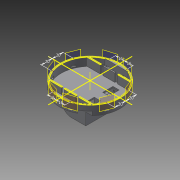
# Autodesk Inventor part: base
Saved by Autodesk Inventor 2014 (Build 180170000, 170)
## iProperties
Created: 2013-06-26
Part Number: base
Material: Generisch
Document SubType Name: Modeling
Designer: hanse
Density: 1 g/cm^3
Appearance: Vorgabe
Author: hanse
Autodesk Inventor part; units mm, degrees
ref_plane "YZ Plane" through (0, 0, 0) normal (1, 0, 0) x (0, 1, 0)
ref_plane "XZ Plane" through (0, 0, 0) normal (0, 1, 0) x (-1, 0, 0)
ref_plane "XY Plane" through (0, 0, 0) normal (0, 0, 1) x (1, 0, 0)
sketch "Skizze1" plane through (0, 0, 0) normal (0, 0, 1) x (1, 0, 0)
  line L0 (29, -20.75) -> (-29, -20.75) projected
  line L1 (29, 20.75) -> (29, -20.75) projected
  line L2 (-29, 20.75) -> (29, 20.75) projected
  line L3 (-29, -20.75) -> (-29, 20.75) projected
  line L4 (4, 34.75) -> (14, 34.75) projected
  line L5 (40.5, 34.75) -> (14, 34.75) projected
  line L6 (14, -34.75) -> (40.5, -34.75) projected
  line L7 (14, -34.75) -> (4, -34.75) projected
  line L8 (40.5, -34.75) -> (40.5, -21.05) projected
  line L9 (40.5, -21.05) -> (40.5, -7.75) projected
  line L10 (40.5, 21.05) -> (40.5, 7.75) projected
  line L11 (40.5, 34.75) -> (40.5, 21.05) projected
  line L12 (4, 34.75) -> (4, 21.05)
  line L13 (4, -34.75) -> (4, -21.05)
  line L14 (13.5, 17.844) -> (13.5, 38.186)
  line L15 (13.5, -17.844) -> (13.5, -38.186)
  line L16 (0, 0) -> (29, 0)
  line L17 (13.5, 17.844) -> (13.5, -17.844)
  line L18 (-15.5, 46.05) -> (42.5, 46.05) projected
  line L19 (42.5, 38.05) -> (-15.5, 38.05) projected
  line L20 (-15.5, -38.05) -> (42.5, -38.05) projected
  line L21 (42.5, -46.05) -> (-15.5, -46.05) projected
  circle A0 centre (13.5, 0) radius 55
  line L22 (40.5, -7.75) -> (29, -7.75)
  line L23 (29, -7.75) -> (29, -26.5586)
  line L24 (29, -26.5586) -> (40.5, -26.5586)
  line L25 (40.5, -26.5586) -> (40.5, -7.75)
  line L26 (40.5, 7.75) -> (40.5, 26.6995)
  line L27 (40.5, 26.6995) -> (29, 26.6995)
  line L28 (29, 26.6995) -> (29, 7.75)
  line L29 (40.5, 7.75) -> (38.25, 7.75) projected
  line L30 (38.25, 7.75) -> (31.25, 7.75) projected
  line L31 (31.25, 7.75) -> (29, 7.75) projected
  line L32 (40.5, 7.75) -> (29, 7.75)
  line L33 (-27.4199, 36.75) -> (54.4199, 36.75)
  line L34 (-27.4199, -36.75) -> (54.4199, -36.75)
  dimension "d0" = 2
  dimension "d1" = 2
  dimension "d22" = 110
  constraints: 32 end point, 5 parallel, 4 point on circle, 4 vertical, 3 collinear, 3 point on line, 2 midpoint, 2 perpendicular, 1 centre point, 1 horizontal, 6 other
  measures "d0" distance between parallel lines of L5 L33
  measures "d1" distance between parallel lines of L6 L34
  measures "d22" diameter of A0
ref_plane "Arbeitsebene1" through (30, 21.05, 2.35) normal (0, 0, 1) x (1, 0, 0)
extrude "Extrusion1" add sketch "Skizze1" along normal up to surface (2.35 mm away) contours L23 L24 L8 L6 L7 L15 L0 | L0 L15 L17 L16 L1 | L15 L34 A0 L33 L14 L2 L3 L0 | L0 L3 L2 L14 L17 L15 | L1 L31 L30 L29 L10 L11 L5 L4 L14 L33 A0 L34 L15 L7 L6 L8 L9 L22 | L16 L17 L14 L2 L1 | L14 L4 L5 L11 L27 L28 L2
sketch "Skizze2" plane through (0, 0, 0) normal (0, 0, -1) x (-1, 0, 0)
  line L0 (-29, 26.6995) -> (-29, 7.75) projected
  line L1 (-29, 7.75) -> (-40.5, 7.75) projected
  line L2 (-40.5, 7.75) -> (-40.5, 26.6995) projected
  line L3 (-40.5, 26.6995) -> (-29, 26.6995) projected
  line L4 (-40.5, -26.5586) -> (-40.5, -7.75) projected
  line L5 (-40.5, -7.75) -> (-29, -7.75) projected
  line L6 (-29, -7.75) -> (-29, -26.5586) projected
  line L7 (-29, -26.5586) -> (-40.5, -26.5586) projected
  line L8 (-54.4199, 36.75) -> (27.4199, 36.75) projected
  line L9 (27.4199, -36.75) -> (-54.4199, -36.75) projected
  line L10 (-29, -20.75) -> (29, -20.75) projected
  line L11 (29, 20.75) -> (-29, 20.75) projected
  line L12 (-42.5, 36.75) -> (-42.5, -36.75)
  line L13 (-29, 7.75) -> (-29, -7.75)
  line L14 (1, 36.75) -> (1, 20.75)
  line L15 (1, -20.75) -> (1, -36.75)
  line L16 (-4, 34.75) -> (-4, 21.05)
  line L17 (-4, -34.75) -> (-4, -21.05)
  point P0 (0, 0)
  dimension "d4" = 2
  dimension "d5" = 5
  constraints: 12 end point, 6 point on line, 3 perpendicular, 2 collinear, 2 vertical, 4 other
  measures "d4" distance between parallel lines of L2 L12
  measures "d5" distance between parallel lines of L14 L16
ref_plane "Arbeitsebene2" through (14, 21.05, -20) normal (0, 0, -1) x (0, 1, 0)
extrude "Extrusion2" add sketch "Skizze2" along normal up to surface (20 mm away) contours L3 L2 L1 L13 L5 L4 L7 L6 L10 L15 L9 L12 L8 L14 L11 L0
sketch "Skizze3" plane through (-1, 20.75, 0) normal (0, -1, 0) x (1, 0, 0)
  line L0 (0, -20) -> (30, -20) projected
  line L1 (30, 0) -> (30, -20) projected
  line L2 (0, 0) -> (30, 0) projected
  line L3 (30, -20) -> (41.5, -20) projected
  line L4 (41.5, -20) -> (30, -20)
  line L5 (30, -20) -> (30, 0)
  line L6 (30, 0) -> (41.5, 0)
  line L7 (41.5, 0) -> (41.5, -20)
  arc A0 (15, 0) -> (15, -20) centre (15, -10) ccw projected
  point P0 (1, 0)
  constraints: 8 end point, 2 parallel, 1 horizontal, 1 perpendicular
ref_plane "Arbeitsebene3" through (4, 34.75, -20) normal (0, 1, 0) x (0, 0, 1)
extrude "Extrusion3" cut sketch "Skizze3" against normal up to surface (14 mm away) contours L1 L6 L7 L3
sketch "Skizze4" plane through (14, 34.75, 0) normal (0, -1, 0) x (1, 0, 0)
  circle A0 centre (8.9, -11.9) radius 1.5 projected
  circle A1 centre (-0.5, -10) radius 2.5 projected
  circle A2 centre (15.5, -6.5) radius 1.5 projected
  point P0 (-14, 0)
extrude "Extrusion4" cut sketch "Skizze4" against normal blind 0.5
sketch "Skizze5" plane through (14, 34.75, -20) normal (0, -1, 0) x (1, 0, 0)
  circle A0 centre (-0.5, 10) radius 1.5 projected
  point P0 (-14, 20)
extrude "Extrusion5" cut sketch "Skizze5" against normal through all
mirror "Spiegeln1" about plane through (0, 0, 0) normal (0, 1, 0) of "Extrusion5", "Extrusion3"
sketch "Skizze6" plane through (14, -34.75, 0) normal (0, 1, 0) x (1, 0, 0)
  circle A0 centre (15.5, 13.5) radius 1.5 projected
  circle A1 centre (8.9, 8.1) radius 1.5 projected
  circle A2 centre (-0.5, 10) radius 2.5 projected
  point P0 (-14, 0)
extrude "Extrusion6" cut sketch "Skizze6" against normal blind 0.5
sketch "Skizze7" plane through (42.5, 36.75, -20) normal (0, 0, -1) x (-1, 0, 0)
  line L0 (43.5, -73.5) -> (0, -73.5)
  line L1 (0, -73.5) -> (0, 0)
  line L2 (0, 0) -> (43.5, 0)
  line L3 (43.5, 0) -> (43.5, -73.5)
  point P0 (42.5, -36.75)
  constraints: 8 end point, 2 parallel, 1 horizontal, 1 perpendicular
extrude "Extrusion7" add sketch "Skizze7" along normal blind 2
sketch "Skizze8" plane through (42.5, 36.75, -22) normal (0, 0, -1) x (-1, 0, 0)
  line L0 (43.5, -73.5) -> (43.5, 0) projected
  line L1 (71.5, -16) -> (13.5, -16) projected
  line L2 (13.5, -57.5) -> (71.5, -57.5) projected
  line L3 (13.5, -16) -> (43.5, -16)
  line L4 (43.5, -16) -> (43.5, -57.5)
  line L5 (43.5, -57.5) -> (13.5, -57.5)
  line L6 (13.5, -57.5) -> (13.5, -16)
  line L7 (11.25, -12.5) -> (11.25, -29) projected
  line L8 (4.25, -29) -> (11.25, -29) projected
  line L9 (4.25, -12.5) -> (4.25, -29) projected
  line L10 (11.25, -12.5) -> (4.25, -12.5) projected
  line L11 (11.25, -61) -> (4.25, -61) projected
  line L12 (4.25, -61) -> (4.25, -44.5) projected
  line L13 (11.25, -44.5) -> (4.25, -44.5) projected
  line L14 (11.25, -61) -> (11.25, -44.5) projected
  line L15 (13.5, -44.5) -> (13.5, -63.3086) projected
  line L16 (13.5, -63.3086) -> (2, -63.3086) projected
  line L17 (2, -63.3086) -> (2, -44.5) projected
  line L18 (2, -44.5) -> (13.5, -44.5) projected
  line L19 (2, -10.0505) -> (13.5, -10.0505) projected
  line L20 (13.5, -10.0505) -> (13.5, -29) projected
  line L21 (13.5, -29) -> (2, -29) projected
  line L22 (2, -29) -> (2, -10.0505) projected
  point P0 (42.5, -36.75)
  constraints: 8 end point, 2 parallel, 2 point on line, 1 horizontal, 1 perpendicular
extrude "Extrusion8" cut sketch "Skizze8" against normal up to next
fillet "Rundung1" radius 17 2 edges at (-1, 28.75, -22) (-1, -28.75, -22)
sketch "Skizze9" plane through (-27.4199, 36.75, 2.35) normal (0, 0, 1) x (1, 0, 0)
  line L0 (0, 0) -> (81.8398, 0) projected
  arc A0 (0, 0) -> (0, -73.5) centre (40.9199, -36.75) ccw projected
  line L1 (81.8398, -73.5) -> (0, -73.5) projected
  arc A1 (81.8398, -73.5) -> (81.8398, 0) centre (40.9199, -36.75) ccw projected
  arc A2 (0.9019, -2) -> (0.9019, -71.5) centre (40.9199, -36.75) ccw
  line L2 (0.9019, -2) -> (80.9379, -2)
  arc A3 (80.9379, -71.5) -> (80.9379, -2) centre (40.9199, -36.75) ccw
  line L3 (80.9379, -71.5) -> (0.9019, -71.5)
  line L4 (0, 0) -> (0, -3.0667)
  line L5 (0, -70.4333) -> (0, -73.5)
  line L6 (81.8398, -73.5) -> (81.8398, -70.4333)
  line L7 (81.8398, 0) -> (81.8398, -3.0667)
  line L8 (0, -2) -> (81.8398, -2)
  line L9 (0, -71.5) -> (81.8398, -71.5)
  circle A4 centre (40.9199, -36.75) radius 55
  line L10 (11.9199, 9.3) -> (69.9199, 9.3) projected
  line L11 (69.9199, -82.8) -> (11.9199, -82.8) projected
  line L12 (15.0762, -85.3) -> (66.7636, -85.3)
  line L13 (15.0762, 11.8) -> (66.7636, 11.8)
  point P0 (27.4199, -36.75)
  dimension "d23" = 2
  dimension "d24" = 2
  dimension "d25" = 2
  dimension "d140" = 2.5
  dimension "d141" = 2.5
  constraints: 20 end point, 12 point on circle, 4 perpendicular, 4 point on line, 3 centre point, 2 equal length, 2 horizontal, 1 coincident, 1 concentric, 3 other
  measures "d23" radial gap between concentric circles of A0 A2
  measures "d24" distance between parallel lines of L9 L1
  measures "d25" distance between parallel lines of L8 L0
  measures "d140" distance between parallel lines of L10 L13
  measures "d141" distance between parallel lines of L11 L12
extrude "Extrusion9" add sketch "Skizze9" along normal blind 5 contours L4 A2 L5 A0 | L0 L7 L8 L2 L4 | A1 L6 A3 L7 | L5 L9 L3 L6 L1 | A4 L13 | L12 A4
sketch "Skizze11" plane through (-27.4199, 36.75, 7.35) normal (0, 0, 1) x (1, 0, 0)
  line L0 (0, -2) -> (81.8398, -2) projected
  line L1 (81.8398, -2) -> (81.8398, -3.0667) projected
  arc A0 (81.8398, -70.4333) -> (81.8398, -3.0667) centre (40.9199, -36.75) ccw projected
  line L2 (81.8398, -70.4333) -> (81.8398, -71.5) projected
  line L3 (81.8398, -71.5) -> (0, -71.5) projected
  line L4 (0, -71.5) -> (0, -70.4333) projected
  arc A1 (0, -3.0667) -> (0, -70.4333) centre (40.9199, -36.75) ccw projected
  line L5 (0, -3.0667) -> (0, -2) projected
  arc A2 (0, 0) -> (0, -73.5) centre (40.9199, -36.75) ccw projected
  line L6 (0, -73.5) -> (81.8398, -73.5) projected
  arc A3 (81.8398, -73.5) -> (81.8398, 0) centre (40.9199, -36.75) ccw projected
  line L7 (81.8398, 0) -> (0, 0) projected
  circle A4 centre (40.9199, -36.75) radius 53
  circle A5 centre (40.9199, -36.75) radius 55
  line L8 (15.0762, 11.8) -> (66.7636, 11.8) projected
  line L9 (66.7636, -85.3) -> (15.0762, -85.3) projected
  line L10 (19.662, 11.8) -> (62.1778, 11.8)
  line L11 (62.1778, -85.3) -> (19.662, -85.3)
  point P0 (27.4199, -36.75)
  constraints: 5 point on circle, 4 end point, 4 point on line, 2 coincident, 1 centre point, 3 other
extrude "Extrusion11" add sketch "Skizze11" along normal blind 10 contours L5 A1 L4 L3 A4 L6 A2 L7 L0 | A4 L7 L0 | A4 L7 A3 L6 L3 L2 A0 L1 L0 | L7 A5 L8 A4 | A4 L8 A5 L7 | L8 A5 A4 | L3 A4 L6 | L6 A4 L9 A5 | L9 A4 A5 | L6 A5 L9 A4
sketch "Skizze23" plane through (-27.4199, 36.75, 7.35) normal (0, 0, 1) x (1, 0, 0)
  arc A0 (19.662, -85.3) -> (62.1778, -85.3) centre (40.9199, -36.75) ccw projected
  line L0 (62.1778, -85.3) -> (19.662, -85.3) projected
  arc A1 (62.1778, 11.8) -> (19.662, 11.8) centre (40.9199, -36.75) ccw projected
  line L1 (19.662, 11.8) -> (62.1778, 11.8) projected
  point P0 (27.4199, -36.75)
extrude "Extrusion19" add sketch "Skizze23" along normal up to surface (10 mm away)
sketch "Skizze12" plane through (13.5, 0, 17.35) normal (0, 0, 1) x (1, 0, 0)
  line L0 (-38.1895, 36.75) -> (38.1895, 36.75) projected
  line L1 (40.9199, -34.75) -> (-40.9199, -34.75) projected
  line L2 (-40.9199, -34.75) -> (-40.9199, -33.6833) projected
  arc A0 (-40.9199, 33.6833) -> (-40.9199, -33.6833) centre (0, 0) ccw projected
  line L3 (-40.9199, 33.6833) -> (-40.9199, 34.75) projected
  line L4 (-40.9199, 34.75) -> (40.9199, 34.75) projected
  line L5 (40.9199, 34.75) -> (40.9199, 33.6833) projected
  arc A1 (40.9199, -33.6833) -> (40.9199, 33.6833) centre (0, 0) ccw projected
  line L6 (40.9199, -33.6833) -> (40.9199, -34.75) projected
  line L7 (-15.9199, 34.75) -> (-15.9199, 36.75)
  line L8 (-15.9199, 36.75) -> (-10.9199, 36.75)
  line L9 (-10.9199, 36.75) -> (-10.9199, 34.75)
  line L10 (-10.9199, 34.75) -> (-15.9199, 34.75)
  line L11 (15.9199, 36.75) -> (10.9199, 36.75)
  line L12 (10.9199, 36.75) -> (10.9199, 34.75)
  line L13 (15.9199, 34.75) -> (10.9199, 34.75)
  line L14 (15.9199, 34.75) -> (15.9199, 36.75)
  point P0 (-13.5, 0)
  dimension "d158" = 25
  dimension "d159" = 25
  dimension "d160" = 5
  dimension "d161" = 5
  constraints: 16 end point, 8 point on line, 4 perpendicular, 2 collinear
  measures "d158" distance between parallel lines of L7 L3
  measures "d159" distance between parallel lines of L14 L5
  measures "d160" distance of L9.end L7.start
  measures "d161" distance of L11.start L11.end
extrude "Extrusion12" cut sketch "Skizze12" against normal up to surface (15 mm away) contours L0 L9 L4 L7 | L4 L5 A1 L6 L1 L2 A0 L3 | L0 L14 L4 L12
mirror "Spiegeln2" about plane through (0, 0, 0) normal (0, 1, 0) of "Extrusion12"
sketch "Skizze13" plane through (13.5, 0, 17.35) normal (0, 0, 1) x (1, 0, 0)
  line L0 (15.9199, -34.75) -> (15.9199, -36.75) projected
  line L1 (38.1895, -36.75) -> (15.9199, -36.75) projected
  arc A0 (-38.1895, -36.75) -> (38.1895, -36.75) centre (0, 0) ccw projected
  line L2 (-15.9199, -36.75) -> (-38.1895, -36.75) projected
  line L3 (-15.9199, -36.75) -> (-15.9199, -34.75) projected
  line L4 (-15.9199, -34.75) -> (-40.9199, -34.75) projected
  line L5 (-40.9199, -34.75) -> (-40.9199, -33.6833) projected
  arc A1 (-40.9199, 33.6833) -> (-40.9199, -33.6833) centre (0, 0) ccw projected
  line L6 (-40.9199, 33.6833) -> (-40.9199, 34.75) projected
  line L7 (-40.9199, 34.75) -> (-15.9199, 34.75) projected
  line L8 (-15.9199, 34.75) -> (-15.9199, 36.75) projected
  line L9 (-38.1895, 36.75) -> (-15.9199, 36.75) projected
  arc A2 (38.1895, 36.75) -> (-38.1895, 36.75) centre (0, 0) ccw projected
  line L10 (15.9199, 36.75) -> (38.1895, 36.75) projected
  line L11 (15.9199, 36.75) -> (15.9199, 34.75) projected
  line L12 (15.9199, 34.75) -> (40.9199, 34.75) projected
  line L13 (40.9199, 34.75) -> (40.9199, 33.6833) projected
  arc A3 (40.9199, -33.6833) -> (40.9199, 33.6833) centre (0, 0) ccw projected
  line L14 (40.9199, -33.6833) -> (40.9199, -34.75) projected
  line L15 (40.9199, -34.75) -> (15.9199, -34.75) projected
  circle A4 centre (0, 0) radius 55 projected
  line L16 (0, 77) -> (0, -77) projected
  line L17 (-77, 0) -> (77, 0) projected
  line L18 (-48.4401, -18.9091) -> (-51.2348, -20)
  line L19 (48.4401, 18.9091) -> (51.2348, 20)
  line L20 (49.3717, -19.2727) -> (51.2348, -20)
  line L21 (-51.2348, 20) -> (-49.3717, 19.2727)
  line L22 (-16, -52.6213) -> (-15.4182, -50.7078)
  line L23 (16, -52.6213) -> (15.4182, -50.7078)
  line L24 (15.4182, 50.7078) -> (16, 52.6213)
  line L25 (-15.4182, 50.7078) -> (-16, 52.6213)
  line L26 (10.9199, -36.75) -> (10.9199, -34.75) projected
  line L27 (10.9199, -34.75) -> (-10.9199, -34.75) projected
  line L28 (-10.9199, -34.75) -> (-10.9199, -36.75) projected
  line L29 (10.9199, -36.75) -> (-10.9199, -36.75) projected
  point P0 (-13.5, 0)
  dimension "d42" = 20
  dimension "d65" = 20
  dimension "d70" = 20
  dimension "d77" = 20
  dimension "d78" = 16
  dimension "d79" = 16
  dimension "d88" = 16
  dimension "d89" = 16
  constraints: 16 end point, 6 point on circle, 5 line through centre, 12 other
  measures "d42" distance from line of L17 L18.end
  measures "d65" distance from line of L17 L19.end
  measures "d70" distance from line of L17 L20.end
  measures "d77" distance from line of L17 L21.start
  measures "d78" distance from line of L25.end L16
  measures "d79" distance from line of L16 L24.end
  measures "d88" distance from line of L16 L22.start
  measures "d89" distance from line of L16 L23.start
ref_plane "Arbeitsebene4" through (-37.7348, -20, 17.35) normal (-0.931541, -0.3636364, 0) x (0.3636364, -0.931541, 0)
ref_plane "Arbeitsebene5" through (-37.7348, 20, 17.35) normal (-0.931541, 0.3636364, 0) x (-0.3636364, -0.931541, 0)
ref_plane "Arbeitsebene6" through (-2.5, 52.6213, 17.35) normal (-0.2909091, 0.9567507, 0) x (-0.9567507, -0.2909091, 0)
ref_plane "Arbeitsebene7" through (29.5, 52.6213, 17.35) normal (0.2909091, 0.9567507, 0) x (-0.9567507, 0.2909091, 0)
ref_plane "Arbeitsebene8" through (64.7348, 20, 17.35) normal (0.931541, 0.3636364, 0) x (-0.3636364, 0.931541, 0)
ref_plane "Arbeitsebene9" through (64.7348, -20, 17.35) normal (0.931541, -0.3636364, 0) x (0.3636364, 0.931541, 0)
ref_plane "Arbeitsebene10" through (29.5, -52.6213, 17.35) normal (0.2909091, -0.9567507, 0) x (0.9567507, 0.2909091, 0)
ref_plane "Arbeitsebene11" through (-2.5, -52.6213, 17.35) normal (-0.2909091, -0.9567507, 0) x (0.9567507, -0.2909091, 0)
sketch "Skizze14" plane through (-37.7348, -20, 17.35) normal (-0.931541, -0.3636364, 0) x (0.3636364, -0.931541, 0)
  line L0 (16.4974, -15) -> (-46.2573, -15) projected
  line L1 (-3.75, -10) -> (3.75, -10)
  line L2 (3.75, -10) -> (3.75, -13)
  line L3 (3.75, -13) -> (-3.75, -13)
  line L4 (-3.75, -13) -> (-3.75, -10)
  line L5 (0, -15) -> (0, 15)
  point P0 (-4.9091, -17.35)
  point P1 (0, 0)
  point P2 (0, 0)
  dimension "d94" = 7.5
  dimension "d95" = 3
  dimension "d97" = 2
  dimension "d100" = 3.75
  constraints: 10 end point, 3 parallel, 1 coincident, 1 horizontal, 1 midpoint, 1 perpendicular, 1 point on line
  measures "d94" distance of L1.start L1.end
  measures "d95" distance of L1.end L2.end
  measures "d97" distance between parallel lines of L0 L3
  measures "d100" distance between parallel lines of L5 L2
extrude "Extrusion16" cut sketch "Skizze14" against normal up to next
sketch "Skizze15" plane through (-37.7348, 20, 17.35) normal (-0.931541, 0.3636364, 0) x (-0.3636364, -0.931541, 0)
  line L0 (-3.75, -10) -> (3.75, -10)
  line L1 (3.75, -10) -> (3.75, -13)
  line L2 (3.75, -13) -> (-3.75, -13)
  line L3 (-3.75, -13) -> (-3.75, -10)
  line L4 (0, -15) -> (0, 15)
  line L5 (46.2573, -15) -> (-16.4974, -15) projected
  point P0 (-6.1364, -17.35)
  point P1 (0, 0)
  point P2 (0, 0)
  dimension "d101" = 7.5
  dimension "d102" = 3
  dimension "d104" = 3.75
  dimension "d129" = 2
  constraints: 10 end point, 3 parallel, 1 coincident, 1 horizontal, 1 midpoint, 1 perpendicular
  measures "d101" distance of L0.start L0.end
  measures "d102" distance of L0.end L1.end
  measures "d104" distance between parallel lines of L4 L1
  measures "d129" distance between parallel lines of L5 L2
extrude "Extrusion17" cut sketch "Skizze15" against normal up to next
sketch "Skizze16" plane through (-2.5, 52.6213, 17.35) normal (-0.2909091, 0.9567507, 0) x (-0.9567507, -0.2909091, 0)
  line L0 (-3.75, -10) -> (3.75, -10)
  line L1 (3.75, -10) -> (3.75, -13)
  line L2 (3.75, -13) -> (-3.75, -13)
  line L3 (-3.75, -13) -> (-3.75, -10)
  line L4 (0, -15) -> (0, 15)
  line L5 (5.1223, -15) -> (29.041, -15) projected
  point P0 (-6.1364, -17.35)
  point P1 (0, 0)
  point P2 (0, 0)
  dimension "d105" = 7.5
  dimension "d106" = 3
  dimension "d108" = 3.75
  dimension "d148" = 2
  constraints: 10 end point, 3 parallel, 1 coincident, 1 horizontal, 1 midpoint, 1 perpendicular
  measures "d105" distance of L0.start L0.end
  measures "d106" distance of L0.end L1.end
  measures "d108" distance between parallel lines of L4 L1
  measures "d148" distance between parallel lines of L2 L5
sketch "Skizze17" plane through (29.5, 52.6213, 17.35) normal (0.2909091, 0.9567507, 0) x (-0.9567507, 0.2909091, 0)
  line L0 (-3.75, -10) -> (3.75, -10)
  line L1 (3.75, -10) -> (3.75, -13)
  line L2 (3.75, -13) -> (-3.75, -13)
  line L3 (-3.75, -13) -> (-3.75, -10)
  line L4 (0, -15) -> (0, 15)
  line L5 (-29.041, -15) -> (-5.1223, -15) projected
  point P0 (-6.1364, -17.35)
  point P1 (0, 0)
  point P2 (0, 0)
  dimension "d109" = 7.5
  dimension "d110" = 3
  dimension "d112" = 3.75
  dimension "d149" = 2
  constraints: 10 end point, 3 parallel, 1 coincident, 1 horizontal, 1 midpoint, 1 perpendicular
  measures "d109" distance of L0.start L0.end
  measures "d110" distance of L0.end L1.end
  measures "d112" distance between parallel lines of L4 L1
  measures "d149" distance between parallel lines of L5 L2
sketch "Skizze18" plane through (64.7348, 20, 17.35) normal (0.931541, 0.3636364, 0) x (-0.3636364, 0.931541, 0)
  line L0 (-3.75, -10) -> (3.75, -10)
  line L1 (3.75, -10) -> (3.75, -13)
  line L2 (3.75, -13) -> (-3.75, -13)
  line L3 (-3.75, -13) -> (-3.75, -10)
  line L4 (0, -15) -> (0, 15)
  line L5 (16.4974, -15) -> (-46.2573, -15) projected
  point P0 (-6.1364, -17.35)
  point P1 (0, 0)
  point P2 (0, 0)
  dimension "d113" = 7.5
  dimension "d114" = 3
  dimension "d116" = 3.75
  dimension "d131" = 2
  constraints: 10 end point, 3 parallel, 1 coincident, 1 horizontal, 1 midpoint, 1 perpendicular
  measures "d113" distance of L0.start L0.end
  measures "d114" distance of L0.end L1.end
  measures "d116" distance between parallel lines of L4 L1
  measures "d131" distance between parallel lines of L2 L5
extrude "Extrusion15" cut sketch "Skizze18" against normal up to next
sketch "Skizze19" plane through (64.7348, -20, 17.35) normal (0.931541, -0.3636364, 0) x (0.3636364, 0.931541, 0)
  line L0 (-3.75, -10) -> (3.75, -10)
  line L1 (3.75, -10) -> (3.75, -13)
  line L2 (3.75, -13) -> (-3.75, -13)
  line L3 (-3.75, -13) -> (-3.75, -10)
  line L4 (0, -15) -> (0, 15)
  line L5 (46.2573, -15) -> (-16.4974, -15) projected
  point P0 (-6.1364, -17.35)
  point P1 (0, 0)
  point P2 (0, 0)
  dimension "d117" = 7.5
  dimension "d118" = 3
  dimension "d120" = 3.75
  dimension "d130" = 2
  constraints: 10 end point, 3 parallel, 1 coincident, 1 horizontal, 1 midpoint, 1 perpendicular
  measures "d117" distance of L0.start L0.end
  measures "d118" distance of L0.end L1.end
  measures "d120" distance between parallel lines of L4 L1
  measures "d130" distance between parallel lines of L2 L5
extrude "Extrusion14" cut sketch "Skizze19" against normal up to next
sketch "Skizze20" plane through (29.5, -52.6213, 17.35) normal (0.2909091, -0.9567507, 0) x (0.9567507, 0.2909091, 0)
  line L0 (-3.75, -10) -> (3.75, -10)
  line L1 (3.75, -10) -> (3.75, -13)
  line L2 (3.75, -13) -> (-3.75, -13)
  line L3 (-3.75, -13) -> (-3.75, -10)
  line L4 (0, -15) -> (0, 15)
  line L5 (-20.5567, -15) -> (0.3385, -15) projected
  point P0 (-6.1364, -17.35)
  point P1 (0, 0)
  point P2 (0, 0)
  dimension "d121" = 7.5
  dimension "d122" = 3
  dimension "d124" = 3.75
  dimension "d146" = 2
  constraints: 10 end point, 3 parallel, 1 coincident, 1 horizontal, 1 midpoint, 1 perpendicular
  measures "d121" distance of L0.start L0.end
  measures "d122" distance of L0.end L1.end
  measures "d124" distance between parallel lines of L4 L1
  measures "d146" distance between parallel lines of L5 L2
sketch "Skizze21" plane through (-2.5, -52.6213, 17.35) normal (-0.2909091, -0.9567507, 0) x (0.9567507, -0.2909091, 0)
  line L0 (-3.75, -10) -> (3.75, -10)
  line L1 (3.75, -10) -> (3.75, -13)
  line L2 (3.75, -13) -> (-3.75, -13)
  line L3 (-3.75, -13) -> (-3.75, -10)
  line L4 (0, -15) -> (0, 15)
  line L5 (-29.041, -15) -> (-5.1223, -15) projected
  point P0 (-6.1364, -17.35)
  point P1 (0, 0)
  point P2 (0, 0)
  dimension "d125" = 7.5
  dimension "d126" = 3
  dimension "d128" = 3.75
  dimension "d147" = 2
  constraints: 10 end point, 3 parallel, 1 coincident, 1 horizontal, 1 midpoint, 1 perpendicular
  measures "d125" distance of L0.start L0.end
  measures "d126" distance of L0.end L1.end
  measures "d128" distance between parallel lines of L4 L1
  measures "d147" distance between parallel lines of L2 L5
extrude "Extrusion20" cut sketch "Skizze17" against normal up to next
extrude "Extrusion21" cut sketch "Skizze16" against normal up to next
extrude "Extrusion22" cut sketch "Skizze20" against normal up to next
extrude "Extrusion23" cut sketch "Skizze21" against normal up to next
sketch "Skizze24" plane through (0, 0, 0) normal (0, 0, -1) x (-1, 0, 0)
  line L0 (-42.5, -36.75) -> (-42.5, 36.75) projected
  arc A0 (-54.4199, 33.6833) -> (-54.4199, -33.6833) centre (-13.5, 0) ccw projected
  line L1 (-54.4199, 33.6833) -> (-54.4199, 34.75) projected
  line L2 (-54.4199, -34.75) -> (-54.4199, -33.6833) projected
  line L3 (-54.4199, 34.75) -> (-29.4199, 34.75) projected
  line L4 (-29.4199, -34.75) -> (-54.4199, -34.75) projected
  line L5 (-42.5, 36.75) -> (-42.5, -34.75)
  line L6 (-42.5, -34.75) -> (-54.4199, -34.75)
  line L7 (-42.5, 34.75) -> (-54.4199, 34.75)
  line L8 (-54.4199, 34.75) -> (-54.4199, -34.75)
  point P0 (0, 0)
  constraints: 8 end point, 4 point on line, 2 perpendicular, 1 collinear
extrude "Extrusion24" cut sketch "Skizze24" against normal up to next contours L4 L2 L8 L1 L3 L0
